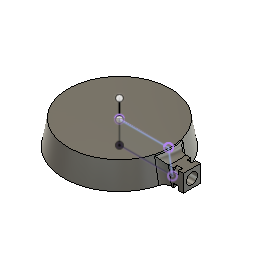
pillow-actuator-v2 (Autodesk Fusion 360 design; units mm, degrees)
Autodesk Fusion 360 part; units mm, degrees
sketch "Sketch1" plane through (0, 0, 0) normal (0, 0, 1) x (1, 0, 0) in component "Pillow Actuator"
  line L0 (0, 0) -> (22.5, 0)
  line L1 (22.5, 0) -> (20.7367, 10)
  line L2 (20.7367, 10) -> (0, 10)
  line L3 (0, 0) -> (0.0175, 0.4)
  line L4 (21.6171, 0.4) -> (19.9949, 9.6)
  line L5 (19.9949, 9.6) -> (0, 9.6)
  line L6 (0, 10) -> (0, 9.6)
  line L7 (21.6171, 0.4) -> (0.0175, 0.4)
  line L8 (0, 0) -> (0, 10) construction
  line L9 (0, 0) -> (0, 15.2884)
  dimension "d15" = 0.4
  dimension "d16" = 80
  dimension "d17" = 0.8
  dimension "d18" = 0.4
  dimension "d19" = 22.5
  dimension "d20" = 10
  constraint coincident L0.start L3.start
  constraint parallel L1 L4
  constraint horizontal L5
  constraint coincident L5.end L8
  constraint coincident L2.end L9
  constraint vertical L9
  measures "d15" distance of L2 L5
  measures "d16" angle of L4 L7
  measures "d17" distance of L1 L4
  measures "d18" distance of L0 L7
  measures "d19" distance of L0.start L0.end
  measures "d20" distance of L0 L2
revolve "Revolve2" add sketch "Sketch1" angle 360 about axis through (0, 0, 0) along (0, 1, 0) contours L0 L1 L2 L3 L4 L5 L6 L7 L9 makes body 1 in component "Pillow Actuator"
ref_plane "WorkPlane1" through (22.5, 0, 0) normal (1, 0, 0) x (0, 1, 0) in component "Pillow Actuator"
sketch "Sketch2" plane through (22.5, 0, 0) normal (1, 0, 0) x (0, 0, -1) in component "Pillow Actuator"
  line L0 (0, 0) -> (-3.5, 0)
  line L1 (-3.5, 0) -> (-3.5, 7)
  line L2 (-3.5, 7) -> (0, 7)
  line L3 (0, 7) -> (0, 0)
  line L4 (3.5, 0) -> (3.5, 7)
  line L5 (3.5, 7) -> (0, 7)
  line L6 (0, 0) -> (3.5, 0)
  dimension "d23" = 7
  dimension "d24" = 3.5
  constraint horizontal L0
  constraint vertical L1
  constraint horizontal L2
  constraint vertical L3
  constraint coincident L0.start L3.end
  constraint symmetric L0.start L3 L6.start
  constraint symmetric L0.end L3 L4.start
  constraint symmetric L1.end L3 L4.end
  constraint symmetric L2.end L3 L5.end
  measures "d23" distance of L0.end L1.end
  measures "d24" distance of L1.end L2.end
extrude "Extrude1" add sketch "Sketch2" along normal mid plane 14 separate body makes body 2 in component "Pillow Actuator"
sketch "Sketch3" plane through (29.5, 0, 0) normal (1, 0, 0) x (0, 0, -1) in component "Pillow Actuator"
  line L0 (-3.5, 0) -> (3.5, 0)
  line L1 (3.5, 0) -> (3.5, 7)
  line L2 (3.5, 7) -> (-3.5, 7)
  line L3 (-3.5, 7) -> (-3.5, 0)
  circle A0 centre (0, 3.5) radius 2.2
  dimension "d28" = 4.4
  measures "d28" diameter of A0
extrude "Extrude2" cut sketch "Sketch3" against normal blind 16 contours A0 bodies 2 1 in component "Pillow Actuator"
ref_plane "WorkPlane2" through (27.5, 3.5, 0) normal (1, 0, 0) x (0, 0, -1) in component "Pillow Actuator"
sketch "Sketch4" plane through (27.5, 3.5, 0) normal (1, 0, 0) x (0, 0, -1) in component "Pillow Actuator"
  circle A0 centre (0, 0) radius 5
  circle A1 centre (0, 0) radius 4
  dimension "d32" = 8
  dimension "d33" = 10
  constraint coincident A0.centre A1.centre
  constraint concentric A0 A1
  measures "d32" diameter of A1
  measures "d33" diameter of A0
extrude "Extrude3" cut sketch "Sketch4" against normal blind 2 bodies 2 in component "Pillow Actuator"
revolve "Revolve3" cut sketch "Sketch1" angle 360 about axis through (0, 0, 0) along (0, 1, 0) contours L3 L4 L5 L7 L9 bodies 2 in component "Pillow Actuator"
combine "Combine2" operation add target body 2 tool bodies 1 in component "Pillow Actuator"
fillet "Fillet1" radius 3 3 edges at (21.5921, 3.5507, -3.5) (21.2657, 7, 0) (21.5921, 3.5507, 3.5) on bodies 2 in component "Pillow Actuator"
sketch "Sketch5" plane through (0, 0, 0) normal (0, 0, 1) x (1, 0, 0) in component "Pillow Actuator"
  line L0 (21.6171, 0.4) -> (19.9949, 9.6)
  line L1 (19.9949, 9.6) -> (0, 9.6)
  line L2 (21.6171, 0.4) -> (0.0175, 0.4)
  line L3 (19.911, 9.5) -> (0, 9.5)
  line L4 (21.498, 0.5) -> (19.911, 9.5)
  line L5 (21.498, 0.5) -> (0.0175, 0.5)
  line L6 (0.0175, 0.4) -> (0.0175, 17)
  dimension "d38" = 0.1
  constraint coincident L2.end L6.start
  constraint perpendicular L5 L6
revolve "Revolve4" add sketch "Sketch5" angle 360 about axis through (0.0175, 0.4, 0) along (0, 1, 0) separate body contours L3 L4 L5 L6 makes body 3 in component "Pillow Actuator"
ref_plane "WorkPlane3" through (20.9482, 0.7818, 2.7182) normal (1, 0, 0) x (0, 0, -1) in component "Pillow Actuator"
sketch "Sketch8" plane through (20.9482, 0.7818, 2.7182) normal (1, 0, 0) x (0, 0, -1) in component "Pillow Actuator"
  circle A0 centre (2.7182, 2.7182) radius 2.2
  circle A1 centre (2.7182, 2.7182) radius 1.875
  dimension "d44" = 3.75
  constraint concentric A0 A1
  measures "d44" diameter of A1
extrude "Extrude4" add sketch "Sketch8" along normal mid plane 2 contours A1 bodies 3 in component "Pillow Actuator"
fillet "Fillet2" radius 1 1 edges at (20.8936, 3.4511, 1.8743) on bodies 3 in component "Pillow Actuator"
component "Pillow Actuator" placed x (1, 0, 0) y (0, 1, 0) z (0, 0, 1) at (3.5894, 4.2686, 0.6423)
equation "Diameter = 45 mm" comment "Outer Diameter"
equation "WallThickness = 0.8 mm"
equation "TopThickness = 0.4 mm"
equation "BottomThickness = 0.4 mm"
equation "Height = 10 mm"
equation "TaperAngle = 80 deg"
equation "d15 = TopThickness"
equation "d16 = TaperAngle"
equation "d17 = WallThickness"
equation "d18 = BottomThickness"
equation "d19 = Diameter / 2"
equation "d20 = Height"
equation "d22 = Diameter / 2"
named bodies: "Actuator", "Support Insert"
